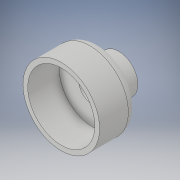
# Autodesk Inventor part: output
Saved by Autodesk Inventor 2019 (Build 230136000, 136)
## iProperties
Created: 2020-03-31
Part Number: output
Material: Generic
Document SubType Name: Modeling
Designer: Bishoy
Density: 1 g/cm^3
Appearance: Default
Author: Bishoy
Autodesk Inventor part; units mm, degrees
ref_plane "YZ Plane" through (0, 0, 0) normal (1, 0, 0) x (0, 1, 0)
ref_plane "XZ Plane" through (0, 0, 0) normal (0, 1, 0) x (-1, 0, 0)
ref_plane "XY Plane" through (0, 0, 0) normal (0, 0, 1) x (1, 0, 0)
sketch "Sketch1" plane through (0, 0, 0) normal (0, 0, 1) x (1, 0, 0)
  circle A0 centre (0, 0) radius 40
  circle A1 centre (0, 0) radius 15
  dimension "d0" = 80
  dimension "d1" = 30
  constraints: 2 centre point, 2 coincident
  measures "d0" diameter of A0
  measures "d1" diameter of A1
extrude "Extrusion1" add sketch "Sketch1" along normal blind 40
sketch "Sketch2" plane through (0, 0, 0) normal (0, 0, -1) x (-1, 0, 0)
  circle A0 centre (0, 0) radius 20
  dimension "d4" = 40
  constraints: 1 centre point, 1 coincident
  measures "d4" diameter of A0
extrude "Extrusion2" add sketch "Sketch2" along normal blind 20
extrude "Extrusion3" cut sketch "Sketch1" against normal blind 20 contours A1
fillet "Fillet1" radius 10 1 edges at (-40, 0, 0)
sketch "Sketch3" plane through (0, 0, 40) normal (0, 0, 1) x (1, 0, 0)
  circle A0 centre (0, 0) radius 35
  dimension "d10" = 70
  constraints: 1 centre point, 1 coincident
  measures "d10" diameter of A0
extrude "Extrusion4" cut sketch "Sketch3" against normal blind 33
body "Solid1"
